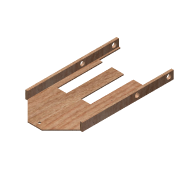
# Autodesk Inventor part: 底板
Saved by Autodesk Inventor 2013 (Build 170138000, 138)
## iProperties
Created: 2012-10-03
Part Number: 底板
Material: 木材(桦木)
Document SubType Name: Modeling
Designer: Zhensheng
Density: 0.55 g/cm^3
Mass: 44.7751 g
Surface Area: 648.48 cm^2
Volume: 81.4092 cm^3
Author: Zhensheng
Autodesk Inventor part; units mm, degrees
ref_plane "YZ Plane" through (0, 0, 0) normal (1, 0, 0) x (0, 1, 0)
ref_plane "XZ Plane" through (0, 0, 0) normal (0, 1, 0) x (-1, 0, 0)
sketch "草图1" plane through (0, 0, 0) normal (0, 0, 1) x (1, 0, 0)
  line L0 (-60, 0) -> (60, 0)
  line L1 (-60, 0) -> (-60, 232)
  line L2 (-60, 232) -> (60, 232)
  line L3 (60, 232) -> (60, 0)
  point P0 (0, 0)
  point P1 (0, 0)
  dimension "宽度" = 120
  dimension "长度" = 232
  dimension "d15" = 120
  constraints: 8 end point, 2 horizontal, 2 vertical, 1 coincident, 1 midpoint
  measures "宽度" distance of L0.start L0.end
  measures "长度" distance of L0.start L1.end
  measures "d15" distance of L1.end L2.end
extrude "拉伸1" add sketch "草图1" along normal blind 2
sketch "草图2" plane through (0, 0, 2) normal (0, 0, 1) x (1, 0, 0)
  line L0 (-60, 0) -> (60, 0) projected
  line L1 (60, 0) -> (60, 232) projected
  line L2 (60, 232) -> (-60, 232) projected
  line L3 (-60, 232) -> (-60, 0) projected
  line L4 (-55, 232) -> (-55, 0)
  line L5 (0, 0) -> (0, 232) construction
  line L6 (55, 0) -> (55, 232)
  dimension "侧厚" = 5
  constraints: 6 end point, 4 point on line, 1 midpoint, 1 other
  measures "侧厚" distance between parallel lines of L4 L3
extrude "拉伸2" add sketch "草图2" along normal blind 15 contours L3 L2 L4 L0 | L6 L2 L1 L0
sketch "草图3" plane through (60, 0, 0) normal (1, 0, 0) x (0, 0, -1)
  line L0 (0, 0) -> (0, 232) projected
  line L1 (0, 232) -> (-17, 232) projected
  line L2 (-17, 0) -> (-17, 232) projected
  line L3 (0, 0) -> (-17, 0) projected
  circle A0 centre (-9.5, 222) radius 5
  circle A1 centre (-9.5, 155.5) radius 5
  line L4 (-9.5, 222) -> (-9.5, 155.5) construction
  point P0 (0, 0)
  dimension "d16" = 10
  dimension "后孔位置" = 10
  dimension "上沿" = 7.5
  dimension "d29" = 10
  dimension "d30" = 66.5
  constraints: 2 centre point, 2 end point
  measures "d16" diameter of A0
  measures "后孔位置" distance from line of L1 L4.start
  measures "上沿" distance from line of L2 L4.start
  measures "d29" diameter of A1
  measures "d30" distance of L4.start L4.end
extrude "拉伸3" cut sketch "草图3" against normal through all contours A0
sketch "草图4" plane through (0, 0, 2) normal (0, 0, 1) x (1, 0, 0)
  line L0 (-52, 232) -> (-52, 187)
  line L1 (-52, 187) -> (52, 187)
  line L2 (52, 187) -> (52, 232)
  line L3 (55, 232) -> (-55, 232)
  line L4 (0, 232) -> (0, 179.736464)
  line L5 (-52, 232) -> (52, 232)
  line L6 (55, 232) -> (55, 0)
  point P0 (0, 0)
  dimension "d26" = 45
  dimension "d39" = 3
  constraints: 10 end point, 1 collinear, 1 horizontal, 1 midpoint, 1 vertical, 1 other
  measures "d26" distance of L1.end L2.end
  measures "d39" distance between parallel lines of L6 L2
extrude "拉伸4" cut sketch "草图4" along normal through all both and the other way through all
extrude "拉伸5" cut sketch "草图3" against normal through all contours A1
sketch "草图5" plane through (0, 0, 2) normal (0, 0, 1) x (1, 0, 0)
  line L0 (-55, 0) -> (-55, 232) projected
  line L1 (-52, 232) -> (-55, 232) projected
  line L2 (-45, 232) -> (-45, 92)
  line L3 (-25, 232) -> (-25, 92)
  line L4 (-45, 92) -> (-25, 92)
  point P0 (0, 0)
  dimension "d33" = 140
  dimension "d34" = 10
  dimension "d35" = 140
  dimension "d36" = 20
  constraints: 6 end point, 2 point on line
  measures "d33" distance of L2.start L2.end
  measures "d34" distance between parallel lines of L2 L0
  measures "d35" distance of L3.start L3.end
  measures "d36" distance between parallel lines of L2 L3
sketch "草图5 outline for 拉伸6" plane through (0, 0, 2) normal (0, 0, 1) x (1, 0, 0)
  line L0 (-45, 232) -> (-25, 232)
  line L1 (-25, 232) -> (-25, 92)
  line L2 (-25, 92) -> (-45, 92)
  line L3 (-45, 92) -> (-45, 232)
extrude "拉伸6" cut sketch "草图5 outline for 拉伸6" along normal through all both and the other way through all
sketch "草图6" plane through (0, 0, 2) normal (0, 0, 1) x (1, 0, 0)
  line L0 (60, 160.5) -> (60, 150.5) projected
  line L1 (55, 150.5) -> (55, 160.5) projected
  line L2 (55, 155.5) -> (0, 155.5) construction
  line L3 (0, 145.5) -> (0, 0) construction
  line L4 (55, 155.5) -> (55, 95.5) construction
  line L5 (55, 95.5) -> (0, 95.5) construction
  line L6 (-10, 95.5) -> (10, 95.5)
  line L7 (52, 187) -> (-25, 187) projected
  line L8 (10, 145.5) -> (10, 177) construction
  line L9 (0, 187) -> (0, 97)
  line L10 (0, 97) -> (20, 97)
  line L11 (20, 97) -> (20, 187)
  dimension "d40" = 60
  dimension "d46" = 90
  dimension "d47" = 20
  dimension "d48" = 10
  constraints: 18 end point, 4 point on line, 3 vertical, 2 horizontal, 1 midpoint, 1 other
  measures "d40" distance of L2.start L4.end
  measures "d46" distance of L9.start L9.end
  measures "d47" distance between parallel lines of L11 L9
  measures "d48" distance between parallel lines of L8 L3
extrude "拉伸7" cut sketch "草图6" against normal through all
sketch "草图7" plane through (0, 0, 2) normal (0, 0, 1) x (1, 0, 0)
  line L0 (60, 227) -> (60, 217) projected
  line L1 (55, 217) -> (55, 227) projected
  line L2 (-60, 232) -> (-60, 0) projected
  line L3 (60, 0) -> (60, 232) projected
  line L4 (-60, 0) -> (60, 0) projected
  line L5 (55, 222) -> (60, 222) construction
  circle A0 centre (0, 10) radius 2.5
  point P0 (0, 0)
  dimension "d49" = 5
  dimension "d50" = 212
  constraints: 2 end point, 1 centre point, 1 midpoint, 1 point on line
  measures "d49" diameter of A0
  measures "d50" distance from line of A0.centre L5
extrude "拉伸8" cut sketch "草图7" against normal through all
sketch "草图8" plane through (0, 0, 2) normal (0, 0, 1) x (1, 0, 0)
  circle A0 centre (0, 10) radius 2.5
  line L0 (20, 187) -> (20, 97)
  line L1 (20, 97) -> (0, 97)
  line L2 (0, 97) -> (0, 187)
  line L3 (0, 187) -> (-25, 187)
  line L4 (-25, 187) -> (-25, 92)
  line L5 (-25, 92) -> (-45, 92)
  line L6 (-45, 92) -> (-45, 187)
  line L7 (-45, 187) -> (-52, 187)
  line L8 (-52, 187) -> (-52, 232)
  line L9 (-52, 232) -> (-55, 232)
  line L10 (-55, 232) -> (-55, 0)
  line L11 (-55, 0) -> (55, 0)
  line L12 (55, 0) -> (55, 232)
  line L13 (55, 232) -> (52, 232)
  line L14 (52, 232) -> (52, 187)
  line L15 (52, 187) -> (20, 187)
  line L16 (-60, 0) -> (-55, 0)
  line L17 (-55, 0) -> (-55, 232)
  line L18 (-55, 232) -> (-60, 232)
  line L19 (-60, 232) -> (-60, 0)
  line L20 (60, 0) -> (60, 232)
  line L21 (60, 232) -> (55, 232)
  line L22 (55, 232) -> (55, 0)
  line L23 (55, 0) -> (60, 0)
  line L24 (-15, 0) -> (-55, 40)
  line L25 (15, 0) -> (55, 40)
  line L26 (0, 0) -> (0, 39.183664) construction
  line L27 (-60, 232) -> (-60, 0)
  line L28 (-55, 40) -> (-60, 40)
  line L29 (-60, 40) -> (-60, 0)
  line L30 (-60, 0) -> (-15, 0)
  line L31 (15, 0) -> (60, 0)
  line L32 (55, 40) -> (60, 40)
  line L33 (60, 0) -> (60, 40)
  dimension "d53" = 30
  dimension "d55" = 40
  constraints: 18 end point, 6 point on line, 1 vertical, 1 other
  measures "d53" distance of L25.start L24.start
  measures "d55" distance from line of L11 L24.end
extrude "拉伸9" cut sketch "草图8" along normal through all both and the other way through all contours L32 L20 L23 L12 | L12 L11 L25 | L11 L10 L24 | L16 L19 L28 L10
ref_plane "工作平面1" through (31, 232, 17) normal (1, 0, 0) x (0, 0, -1)
sketch "草图9" plane through (31, 232, 17) normal (1, 0, 0) x (0, 0, -1)
  line L0 (17, -192) -> (17, 0)
  line L1 (17, -56.209089) -> (-323, -175.94833)
  line L2 (-322.950917, -180.94833) -> (17, -61.209089)
  line L3 (17, -56.209089) -> (17, -61.209089)
  line L4 (-322.950917, -180.94833) -> (-323, -175.94833)
  point P0 (17, -232)
  dimension "d59" = 340
  dimension "d64" = 5
  dimension "d65" = 5
  constraints: 8 end point, 1 collinear
  measures "d59" distance from line of L0 L1.end
  measures "d64" distance of L2.end L1.start
  measures "d65" vertical distance of L2.start L1.end
extrude "拉伸11" [suppressed]
